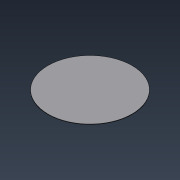
# Autodesk Inventor part: Papier 50mm
Saved by Autodesk Inventor 2022.1 (Build 261234020, 234B)
## iProperties
Created: 2015-09-03
Part Number: Papier 50mm
Material: Allgemein
Document SubType Name: Modeling
Designer: ryll
Density: 1 g/cm^3
Appearance: Vorgabe
Mass: 0.490874 g
Surface Area: 39.6626 cm^2
Volume: 0.490874 cm^3
Author: ryll
Autodesk Inventor part; units mm, degrees
ref_plane "YZ Plane" through (0, 0, 0) normal (1, 0, 0) x (0, 1, 0)
ref_plane "XZ Plane" through (0, 0, 0) normal (0, 1, 0) x (-1, 0, 0)
ref_plane "XY Plane" through (0, 0, 0) normal (0, 0, 1) x (1, 0, 0)
sketch "Skizze1" plane through (0, 0, 0) normal (0, 0, 1) x (1, 0, 0)
  line L0 (0, 35) -> (0, -35) projected
  line L1 (-35, 0) -> (35, 0) projected
  circle A0 centre (0, 0) radius 25
  dimension "d4" = 50
  constraints: 2 midpoint, 1 centre point
  measures "d4" diameter of A0
extrude "Extrusion1" add sketch "Skizze1" along normal blind 0.25
